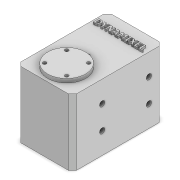
# Autodesk Inventor part: DummyDynamixel
Saved by Autodesk Inventor 2021 (Build 250183000, 183)
## iProperties
Created: 2022-10-19
Part Number: DummyDynamixel
Material: Generic
Document SubType Name: Modeling
Designer: alyn649
Density: 1 g/cm^3
Appearance: Default
Author: alyn649
Autodesk Inventor part; units mm, degrees
ref_plane "YZ Plane" through (0, 0, 0) normal (1, 0, 0) x (0, 1, 0)
ref_plane "XZ Plane" through (0, 0, 0) normal (0, 1, 0) x (-1, 0, 0)
ref_plane "XY Plane" through (0, 0, 0) normal (0, 0, 1) x (1, 0, 0)
sketch "Sketch1" plane through (0, 0, 0) normal (0, 1, 0) x (-1, 0, 0)
  line L0 (14.25, -23.25) -> (-14.25, -23.25)
  line L1 (-14.25, -23.25) -> (-14.25, 23.25)
  line L2 (-14.25, 23.25) -> (14.25, 23.25)
  line L3 (14.25, 23.25) -> (14.25, -23.25)
  point P0 (0, 0)
  point P1 (14.25, 0)
  point P2 (0, -23.25)
  dimension "d1" = 28.5
  dimension "d2" = 46.5
  constraints: 8 end point, 2 midpoint, 2 parallel, 1 horizontal, 1 horizontal alignment, 1 perpendicular, 1 vertical alignment
  measures "d1" distance of L0.start L0.end
  measures "d2" distance of L2.end L0.start
extrude "Extrusion1" add sketch "Sketch1" along normal blind 34
chamfer "Chamfer1" distance 2 angle 45 4 edges at (-14.25, 17, -23.25) (14.25, 17, -23.25) (14.25, 17, 23.25) (-14.25, 17, 23.25)
sketch "Sketch2" plane through (0, 34, 0) normal (0, 1, 0) x (1, 0, 0)
  circle A0 centre (0, -12) radius 9.75
  line L0 (-12.25, -23.25) -> (12.25, -23.25) projected
  point P0 (0, 0)
  dimension "d8" = 19.5
  dimension "d9" = 11.25
  constraints: 1 centre point, 1 vertical alignment
  measures "d8" diameter of A0
  measures "d9" distance from line of A0.centre L0
extrude "Extrusion2" add sketch "Sketch2" along normal blind 2
sketch "Sketch3" plane through (0, 0, 0) normal (0, -1, 0) x (1, 0, 0)
  line L0 (10.75, -19.75) -> (-10.75, -19.75)
  line L1 (-10.75, -19.75) -> (-10.75, 19.75)
  line L2 (-10.75, 19.75) -> (10.75, 19.75)
  line L3 (10.75, 19.75) -> (10.75, -19.75)
  line L4 (12.25, -23.25) -> (-12.25, -23.25) projected
  line L5 (14.25, 21.25) -> (14.25, -21.25) projected
  point P0 (0, 0)
  point P1 (0, -19.75)
  point P2 (10.75, 0)
  dimension "d12" = 3.5
  dimension "d13" = 3.5
  constraints: 8 end point, 2 midpoint, 2 parallel, 1 horizontal, 1 horizontal alignment, 1 perpendicular, 1 vertical alignment
  measures "d12" distance between parallel lines of L4 L0
  measures "d13" distance between parallel lines of L5 L3
extrude "Extrusion3" cut sketch "Sketch3" against normal blind 31
sketch "Sketch4" plane through (-14.25, 0, -21.25) normal (-1, 0, 0) x (0, 0, 1)
  line L0 (29.25, 11) -> (5.25, 11) construction
  line L1 (5.25, 11) -> (5.25, 23) construction
  line L2 (5.25, 23) -> (29.25, 23) construction
  line L3 (29.25, 23) -> (29.25, 11) construction
  line L4 (0, 34) -> (42.5, 34) construction
  line L5 (44.5, 0) -> (44.5, 34) construction
  circle A0 centre (29.25, 23) radius 1.35
  circle A1 centre (5.25, 23) radius 1.35
  circle A2 centre (5.25, 11) radius 1.35
  circle A3 centre (29.25, 11) radius 1.35
  point P0 (21.25, 0)
  dimension "d16" = 24
  dimension "d17" = 12
  dimension "d18" = 11
  dimension "d19" = 15.25
  dimension "d20" = 2.7
  dimension "d21" = 2.7
  dimension "d22" = 2.7
  dimension "d23" = 2.7
  constraints: 8 end point, 4 centre point, 4 coincident, 2 parallel, 1 horizontal, 1 perpendicular
  measures "d16" distance of L0.start L0.end
  measures "d17" distance of L0.end L1.end
  measures "d18" distance between parallel lines of L4 L2
  measures "d19" distance from line of L5 L2.end
  measures "d20" diameter of A2
  measures "d21" diameter of A1
  measures "d22" diameter of A0
  measures "d23" diameter of A3
extrude "Extrusion4" cut sketch "Sketch4" against normal up to surface (3.5 mm away)
sketch "Sketch5" plane through (12.25, 0, -23.25) normal (0, 0, -1) x (-1, 0, 0)
  circle A0 centre (20.25, 11) radius 1.35
  circle A1 centre (20.25, 23) radius 1.35
  line L0 (0, 34) -> (24.5, 34) projected
  line L1 (26.5, 0) -> (26.5, 34) projected
  point P0 (12.25, 0)
  dimension "d26" = 12
  dimension "d27" = 11
  dimension "d28" = 6.25
  dimension "d29" = 2.7
  dimension "d30" = 2.7
  constraints: 2 centre point, 1 vertical alignment
  measures "d26" distance of A1.centre A0.centre
  measures "d27" distance from line of L0 A1.centre
  measures "d28" distance from line of L1 A1.centre
  measures "d29" diameter of A0
  measures "d30" diameter of A1
extrude "Extrusion5" cut sketch "Sketch5" against normal up to surface (3.5 mm away)
sketch "Sketch6" plane through (-10.75, 0, 19.75) normal (1, 0, 0) x (0, 0, -1)
  circle A0 centre (35.75, 23) radius 1.35 construction
  circle A1 centre (35.75, 11) radius 1.35 construction
  circle A2 centre (11.75, 11) radius 1.35 construction
  circle A3 centre (11.75, 23) radius 1.35 construction
  line L0 (35.75, 25.829) -> (38.2, 24.4145)
  line L1 (38.2, 24.4145) -> (38.2, 21.5855)
  line L2 (38.2, 21.5855) -> (35.75, 20.171)
  line L3 (35.75, 20.171) -> (33.3, 21.5855)
  line L4 (33.3, 21.5855) -> (33.3, 24.4145)
  line L5 (33.3, 24.4145) -> (35.75, 25.829)
  line L6 (35.75, 13.829) -> (38.2, 12.4145)
  line L7 (38.2, 12.4145) -> (38.2, 9.5855)
  line L8 (38.2, 9.5855) -> (35.75, 8.171)
  line L9 (35.75, 8.171) -> (33.3, 9.5855)
  line L10 (33.3, 9.5855) -> (33.3, 12.4145)
  line L11 (33.3, 12.4145) -> (35.75, 13.829)
  line L12 (11.75, 25.829) -> (14.2, 24.4145)
  line L13 (14.2, 24.4145) -> (14.2, 21.5855)
  line L14 (14.2, 21.5855) -> (11.75, 20.171)
  line L15 (11.75, 20.171) -> (9.3, 21.5855)
  line L16 (9.3, 21.5855) -> (9.3, 24.4145)
  line L17 (9.3, 24.4145) -> (11.75, 25.829)
  line L18 (11.75, 13.829) -> (14.2, 12.4145)
  line L19 (14.2, 12.4145) -> (14.2, 9.5855)
  line L20 (14.2, 9.5855) -> (11.75, 8.171)
  line L21 (11.75, 8.171) -> (9.3, 9.5855)
  line L22 (9.3, 9.5855) -> (9.3, 12.4145)
  line L23 (9.3, 12.4145) -> (11.75, 13.829)
  point P0 (19.75, 0)
  dimension "d34" = 4.9
  dimension "d35" = 4.9
  dimension "d36" = 4.9
  dimension "d37" = 4.9
  constraints: 48 end point, 4 coincident, 52 other
  measures "d34" distance between parallel lines of L1 L4
  measures "d35" distance between parallel lines of L7 L10
  measures "d36" distance between parallel lines of L13 L16
  measures "d37" distance between parallel lines of L19 L22
extrude "Extrusion6" cut sketch "Sketch6" against normal blind 1.8
sketch "Sketch7" plane through (-10.75, 0, -19.75) normal (0, 0, 1) x (1, 0, 0)
  circle A0 centre (2.75, 23) radius 1.35 construction
  circle A1 centre (2.75, 11) radius 1.35 construction
  line L0 (2.75, 25.829) -> (5.2, 24.4145)
  line L1 (5.2, 24.4145) -> (5.2, 21.5855)
  line L2 (5.2, 21.5855) -> (2.75, 20.171)
  line L3 (2.75, 20.171) -> (0.3, 21.5855)
  line L4 (0.3, 21.5855) -> (0.3, 24.4145)
  line L5 (0.3, 24.4145) -> (2.75, 25.829)
  line L6 (2.75, 13.829) -> (5.2, 12.4145)
  line L7 (5.2, 12.4145) -> (5.2, 9.5855)
  line L8 (5.2, 9.5855) -> (2.75, 8.171)
  line L9 (2.75, 8.171) -> (0.3, 9.5855)
  line L10 (0.3, 9.5855) -> (0.3, 12.4145)
  line L11 (0.3, 12.4145) -> (2.75, 13.829)
  point P0 (10.75, 0)
  dimension "d40" = 4.9
  dimension "d41" = 4.9
  constraints: 24 end point, 2 coincident, 26 other
  measures "d40" distance between parallel lines of L1 L4
  measures "d41" distance between parallel lines of L7 L10
extrude "Extrusion7" cut sketch "Sketch7" against normal blind 1.8
mirror "Mirror1" about plane through (0, 0, 0) normal (1, 0, 0) of "Extrusion4", "Extrusion5", "Extrusion6", "Extrusion7"
sketch "Sketch8" plane through (0, 36, 12) normal (0, 1, 0) x (1, 0, 0)
  circle A0 centre (-5.6569, 5.6569) radius 0.9
  circle A1 centre (0, 0) radius 9.75 construction
  circle A2 centre (-5.6569, -5.6569) radius 0.9
  circle A3 centre (5.6569, -5.6569) radius 0.9
  circle A4 centre (5.6569, 5.6569) radius 0.9
  line L0 (0, 0) -> (-2.0555, 0) construction
  line L1 (0, 0) -> (-5.6569, 5.6569) construction
  point P0 (0, 12)
  dimension "d44" = 8
  dimension "d45" = 1.8
  dimension "d48" = 360
  dimension "d50" = 45
  constraints: 4 centre point, 4 end point, 1 horizontal, 9 other
  measures "d44" distance of L0.start L1.end
  measures "d45" diameter of A0
  measures "d50" angle of L1 L0
extrude "Extrusion8" cut sketch "Sketch8" against normal up to surface (5 mm away)
sketch "Sketch9" plane through (0, 34, 0) normal (0, 1, 0) x (1, 0, 0)
  line L0 (-12.8099, 16.9998) -> (9.4252, 16.9998) construction
  line L1 (9.4252, 16.9998) -> (9.4252, 14.1415) construction
  line L2 (9.4252, 14.1415) -> (-12.8099, 14.1415) construction
  line L3 (-12.8099, 14.1415) -> (-12.8099, 16.9998) construction
  spline S0 degree 2 poles (-9.7722, 15.5682) (-9.7722, 15.1406) (-10.1455, 14.4683) (-10.4297, 14.2879) knots 0 0 0 1 2 2 2
  spline S1 degree 2 poles (-10.4297, 14.2879) (-10.667, 14.1346) (-11.2256, 14.0456) (-11.5395, 14.0456) knots 0 0 0 1 2 2 2
  line L4 (-11.5395, 14.0456) -> (-12.4935, 14.0456)
  line L5 (-12.4935, 14.0456) -> (-12.4935, 17.0956)
  line L6 (-12.4935, 17.0956) -> (-11.5493, 17.0956)
  spline S2 degree 2 poles (-11.5493, 17.0956) (-11.228, 17.0956) (-10.667, 17.0141) (-10.4198, 16.8559) knots 0 0 0 1 2 2 2
  spline S3 degree 2 poles (-10.4198, 16.8559) (-10.1207, 16.6631) (-9.7722, 16.0106) (-9.7722, 15.5682) knots 0 0 0 1 2 2 2
  spline S4 degree 2 poles (-10.5582, 15.5731) (-10.5582, 15.8747) (-10.7658, 16.3047) (-10.9784, 16.4258) knots 0 0 0 1 2 2 2
  spline S5 degree 2 poles (-10.9784, 16.4258) (-11.1341, 16.5099) (-11.4752, 16.5272) (-11.7125, 16.5272) knots 0 0 0 1 2 2 2
  line L7 (-11.7125, 16.5272) -> (-11.7273, 16.5272)
  line L8 (-11.7273, 16.5272) -> (-11.7273, 14.6166)
  line L9 (-11.7273, 14.6166) -> (-11.7125, 14.6166)
  spline S6 degree 2 poles (-11.7125, 14.6166) (-11.4554, 14.6166) (-11.102, 14.6339) (-10.9413, 14.7352) knots 0 0 0 1 2 2 2
  spline S7 degree 2 poles (-10.9413, 14.7352) (-10.7535, 14.8539) (-10.5582, 15.2716) (-10.5582, 15.5731) knots 0 0 0 1 2 2 2
  line L10 (-6.7816, 17.0956) -> (-7.8345, 15.3185)
  line L11 (-7.8345, 15.3185) -> (-7.8345, 14.0456)
  line L12 (-7.8345, 14.0456) -> (-8.6007, 14.0456)
  line L13 (-8.6007, 14.0456) -> (-8.6007, 15.2815)
  line L14 (-8.6007, 15.2815) -> (-9.6709, 17.0956)
  line L15 (-9.6709, 17.0956) -> (-8.7984, 17.0956)
  line L16 (-8.7984, 17.0956) -> (-8.2027, 16.0081)
  line L17 (-8.2027, 16.0081) -> (-7.6269, 17.0956)
  line L18 (-7.6269, 17.0956) -> (-6.7816, 17.0956)
  line L19 (-3.8922, 14.0456) -> (-4.6288, 14.0456)
  line L20 (-4.6288, 14.0456) -> (-5.8053, 16.1713)
  line L21 (-5.8053, 16.1713) -> (-5.8053, 14.0456)
  line L22 (-5.8053, 14.0456) -> (-6.5047, 14.0456)
  line L23 (-6.5047, 14.0456) -> (-6.5047, 17.0956)
  line L24 (-6.5047, 17.0956) -> (-5.5655, 17.0956)
  line L25 (-5.5655, 17.0956) -> (-4.5917, 15.3482)
  line L26 (-4.5917, 15.3482) -> (-4.5917, 17.0956)
  line L27 (-4.5917, 17.0956) -> (-3.8922, 17.0956)
  line L28 (-3.8922, 17.0956) -> (-3.8922, 14.0456)
  line L29 (-3.6006, 14.0456) -> (-2.5699, 17.0956)
  line L30 (-2.5699, 17.0956) -> (-1.7345, 17.0956)
  line L31 (-1.7345, 17.0956) -> (-0.7038, 14.0456)
  line L32 (-0.7038, 14.0456) -> (-1.4923, 14.0456)
  line L33 (-1.4923, 14.0456) -> (-1.6826, 14.6685)
  line L34 (-1.6826, 14.6685) -> (-2.6416, 14.6685)
  line L35 (-2.6416, 14.6685) -> (-2.8344, 14.0456)
  line L36 (-2.8344, 14.0456) -> (-3.6006, 14.0456)
  line L37 (-1.8506, 15.2221) -> (-2.1621, 16.2306)
  line L38 (-2.1621, 16.2306) -> (-2.476, 15.2221)
  line L39 (-2.476, 15.2221) -> (-1.8506, 15.2221)
  line L40 (2.7145, 14.0456) -> (1.9532, 14.0456)
  line L41 (1.9532, 14.0456) -> (1.9532, 16.0674)
  line L42 (1.9532, 16.0674) -> (1.3996, 14.7624)
  line L43 (1.3996, 14.7624) -> (0.8756, 14.7624)
  line L44 (0.8756, 14.7624) -> (0.3219, 16.0674)
  line L45 (0.3219, 16.0674) -> (0.3219, 14.0456)
  line L46 (0.3219, 14.0456) -> (-0.3998, 14.0456)
  line L47 (-0.3998, 14.0456) -> (-0.3998, 17.0956)
  line L48 (-0.3998, 17.0956) -> (0.4826, 17.0956)
  line L49 (0.4826, 17.0956) -> (1.1598, 15.5904)
  line L50 (1.1598, 15.5904) -> (1.8321, 17.0956)
  line L51 (1.8321, 17.0956) -> (2.7145, 17.0956)
  line L52 (2.7145, 17.0956) -> (2.7145, 14.0456)
  line L53 (4.8648, 14.0456) -> (3.2236, 14.0456)
  line L54 (3.2236, 14.0456) -> (3.2236, 14.5771)
  line L55 (3.2236, 14.5771) -> (3.6611, 14.5771)
  line L56 (3.6611, 14.5771) -> (3.6611, 16.5642)
  line L57 (3.6611, 16.5642) -> (3.2236, 16.5642)
  line L58 (3.2236, 16.5642) -> (3.2236, 17.0956)
  line L59 (3.2236, 17.0956) -> (4.8648, 17.0956)
  line L60 (4.8648, 17.0956) -> (4.8648, 16.5642)
  line L61 (4.8648, 16.5642) -> (4.4273, 16.5642)
  line L62 (4.4273, 16.5642) -> (4.4273, 14.5771)
  line L63 (4.4273, 14.5771) -> (4.8648, 14.5771)
  line L64 (4.8648, 14.5771) -> (4.8648, 14.0456)
  line L65 (7.9543, 14.0456) -> (7.0695, 14.0456)
  line L66 (7.0695, 14.0456) -> (6.4812, 15.017)
  line L67 (6.4812, 15.017) -> (5.8806, 14.0456)
  line L68 (5.8806, 14.0456) -> (5.0329, 14.0456)
  line L69 (5.0329, 14.0456) -> (6.024, 15.5805)
  line L70 (6.024, 15.5805) -> (5.0724, 17.0956)
  line L71 (5.0724, 17.0956) -> (5.9573, 17.0956)
  line L72 (5.9573, 17.0956) -> (6.5084, 16.1737)
  line L73 (6.5084, 16.1737) -> (7.0744, 17.0956)
  line L74 (7.0744, 17.0956) -> (7.9222, 17.0956)
  line L75 (7.9222, 17.0956) -> (6.9657, 15.6127)
  line L76 (6.9657, 15.6127) -> (7.9543, 14.0456)
  line L77 (8.246, 14.0456) -> (8.246, 17.0956)
  line L78 (8.246, 17.0956) -> (10.3073, 17.0956)
  line L79 (10.3073, 17.0956) -> (10.3073, 16.5148)
  line L80 (10.3073, 16.5148) -> (9.0073, 16.5148)
  line L81 (9.0073, 16.5148) -> (9.0073, 15.9785)
  line L82 (9.0073, 15.9785) -> (10.206, 15.9785)
  line L83 (10.206, 15.9785) -> (10.206, 15.3976)
  line L84 (10.206, 15.3976) -> (9.0073, 15.3976)
  line L85 (9.0073, 15.3976) -> (9.0073, 14.6265)
  line L86 (9.0073, 14.6265) -> (10.3073, 14.6265)
  line L87 (10.3073, 14.6265) -> (10.3073, 14.0456)
  line L88 (10.3073, 14.0456) -> (8.246, 14.0456)
  line L89 (12.8605, 14.0456) -> (10.8264, 14.0456)
  line L90 (10.8264, 14.0456) -> (10.8264, 17.0956)
  line L91 (10.8264, 17.0956) -> (11.5926, 17.0956)
  line L92 (11.5926, 17.0956) -> (11.5926, 14.6265)
  line L93 (11.5926, 14.6265) -> (12.8605, 14.6265)
  line L94 (12.8605, 14.6265) -> (12.8605, 14.0456)
  point P0 (0, 0)
  constraints: 2 other
emboss "Emboss1" sketch "Sketch9" operation add depth 1 direction (0, -1, 0)
sketch "Sketch10" plane through (0, 34, 0) normal (0, 1, 0) x (1, 0, 0)
  circle A0 centre (0, -1.25) radius 1
  circle A1 centre (0, -12) radius 9.75 projected
  point P0 (0, 0)
  dimension "d55" = 2
  constraints: 1 centre point, 1 tangent, 1 vertical alignment
  measures "d55" diameter of A0
extrude "Extrusion9" cut sketch "Sketch10" against normal through all contours A0
sketch "Sketch11" plane through (0, 0, 0) normal (1, 0, 0) x (0, 1, 0)
  line L0 (0, -19.75) -> (31, -19.75) construction
  line L1 (31, -19.75) -> (31, 0.25) construction
  line L2 (31, 0.25) -> (34, 0.25) construction
  line L3 (34, 0.25) -> (34, -14.0456) construction
  line L4 (34, -14.0456) -> (35, -14.0456) construction
  line L5 (35, -14.0456) -> (35, -17.0956) construction
  line L6 (35, -17.0956) -> (34, -17.0956) construction
  line L7 (34, -17.0956) -> (34, -23.25) construction
  line L8 (34, -23.25) -> (0, -23.25) construction
  line L9 (0, -23.25) -> (0, -19.75) construction
  line L10 (31, 19.75) -> (0, 19.75) construction
  line L11 (0, 19.75) -> (0, 23.25) construction
  line L12 (0, 23.25) -> (34, 23.25) construction
  line L13 (34, 23.25) -> (34, 21.75) construction
  line L14 (34, 21.75) -> (36, 21.75) construction
  line L15 (36, 21.75) -> (36, 2.25) construction
  line L16 (36, 2.25) -> (34, 2.25) construction
  line L17 (34, 2.25) -> (31, 2.25) construction
  line L18 (31, 2.25) -> (31, 19.75) construction
  circle A0 centre (28, -0.75) radius 1.5
  line L19 (31, -5.75) -> (23, -5.75)
  line L20 (23, -5.75) -> (23, 4.25)
  line L21 (23, 4.25) -> (31, 4.25)
  line L22 (31, 4.25) -> (31, -5.75)
  circle A1 centre (28, -0.75) radius 3 construction
  line L23 (29.1991, 0.75) -> (26.7018, 0.75) construction
  point P0 (0, 0)
  point P1 (23, -0.75)
  dimension "d58" = 3
  dimension "d59" = 6
  dimension "d60" = 0.5
  dimension "d61" = 10
  dimension "d62" = 8
  constraints: 10 end point, 2 centre point, 2 horizontal, 2 parallel, 2 tangent, 1 coincident, 1 horizontal alignment, 1 midpoint, 1 perpendicular, 1 point on line
  measures "d58" diameter of A0
  measures "d59" diameter of A1
  measures "d60" distance between parallel lines of L2 L23
  measures "d61" distance between parallel lines of L19 L21
  measures "d62" distance between parallel lines of L1 L20
extrude "Extrusion10" add sketch "Sketch11" along normal mid plane 8
sketch "Sketch12" plane through (-4, 23, -5.75) normal (0, -1, 0) x (1, 0, 0)
  circle A0 centre (4, 7) radius 1 construction
  line L0 (5, 5.75) -> (3, 5.75)
  line L1 (3, 5.75) -> (3, 10)
  line L2 (3, 10) -> (5, 10)
  line L3 (5, 10) -> (5, 5.75)
  line L4 (0, 10) -> (8, 10) projected
  point P0 (4, 5.75)
  point P1 (4, 10)
  point P2 (4, 5.75)
  constraints: 8 end point, 3 midpoint, 2 parallel, 1 coincident, 1 horizontal, 1 perpendicular, 1 tangent
extrude "Extrusion11" cut sketch "Sketch12" against normal up to surface (8 mm away)
fillet "Fillet1" radius 5 3 edges at (2.5, 23, 4.25) (0, 23, -5.75) (-2.5, 23, 4.25)
equation "\"d13\" = d12"
equation "\"d21\" = d20"
equation "\"d22\" = d21"
equation "\"d23\" = d20"
equation "\"d24\" = d19"
equation "\"d30\" = d29"
equation "\"d35\" = d34"
equation "\"d36\" = d34"
equation "\"d37\" = d36"
equation "\"d41\" = d40"
body "Solid1"
